# Autodesk Inventor part: Synchronous Pulley2
Saved by Autodesk Inventor 2013 (Build 170138000, 138)
## iProperties
Created: 2013-09-28
Part Number: Synchronous Pulley2
Material: Steel
Document SubType Name: Modeling
Designer: Admin
Density: 1 g/cm^3
CustomPartVersion: 1
Author: Admin
Autodesk Inventor part; units mm, degrees
ref_plane "YZ Plane" through (0, 0, 0) normal (1, 0, 0) x (0, 1, 0)
ref_plane "XZ Plane" through (0, 0, 0) normal (0, 1, 0) x (-1, 0, 0)
ref_plane "XY Plane" through (0, 0, 0) normal (0, 0, 1) x (1, 0, 0)
sketch "Pulley Sketch" plane through (0, 0, 0) normal (0, 0, 1) x (1, 0, 0)
  circle A0 centre (0, 0) radius 9.7021 construction
  circle A1 centre (0, 0) radius 9.4481
  circle A2 centre (0, 0) radius 7.7971
  line L0 (-1.3828, 9.3463) -> (-0.6604, 7.7971)
  line L1 (-0.6604, 7.7971) -> (0.6604, 7.7971)
  line L2 (0.6604, 7.7971) -> (1.3828, 9.3463)
  line L3 (0, 0) -> (0, 9.4481) construction
  point P0 (0, 7.7971)
  dimension "d0" = 19.4042
  dimension "d1" = 0.254
  dimension "d2" = 1.651
  dimension "d3" = 50
  dimension "d4" = 1.3208
  constraints: 8 end point, 3 coincident, 3 point on circle, 2 centre point, 1 horizontal, 1 midpoint, 1 point on line, 1 vertical, 1 vertical alignment, 3 other
  measures "d0" diameter of A0
  measures "d1" radial gap between concentric circles of A0 A1
  measures "d3" angle of L2 L0
  measures "d4" distance of L0.end L1.end
extrude "Base Body" add sketch "Pulley Sketch" along normal mid plane 12.54 contours A2 | A1 L0 L1 L2 | L2 L1 L0 A1
extrude "Tooth" cut sketch "Pulley Sketch" along normal through all both and the other way through all contours L2 L1 L0 A1 picked at (0, 8.8902)
fillet "Tooth Fillet" radius 0.4064 2 edges at (0.6604, 7.7971, 0) (-0.6604, 7.7971, 0)
fillet "Tooth Fillet" radius 0.635 4 edges at (-1.3828, 9.3463, 3.135) (-1.3828, 9.3463, -3.135) (1.3828, 9.3463, 3.135) (1.3828, 9.3463, -3.135)
pattern_circular "Teeth" count 12 over 360 about axis through (0, 0, -10) along (0, 0, 1) of "Tooth", "Tooth Fillet"
pulley flange "Left flange" diameter 18.8962 height 3 thickness 1.73 bend angle 10 centre (0, 0, -6.27) toward (0, 0, -1)
pulley flange "Right flange" diameter 18.8962 height 3 thickness 1.73 bend angle 10 centre (0, 0, 6.27) toward (0, 0, 1)
equation "\"d1\" = da_a"
equation "\"d2\" = da_hg"
equation "\"d3\" = 2 * da_fi"
equation "\"d4\" = da_bw"
equation "\"d5\" = da_bf"
equation "\"d7\" = da_bf"
equation "\"d9\" = da_rb"
equation "\"d10\" = da_rt"
equation "\"da_pb\" = 5.08"
equation "\"da_fi\" = 25deg"
equation "\"da_hg\" = 1.651"
equation "\"da_bw\" = 1.3208"
equation "\"da_rb\" = 0.4064"
equation "\"da_rt\" = 0.635"
equation "\"da_a\" = 0.254"
equation "\"da_bf\" = 12.54"
equation "\"da_wf\" = 1.73"
equation "\"da_hf\" = 3"
body "Solid1"
